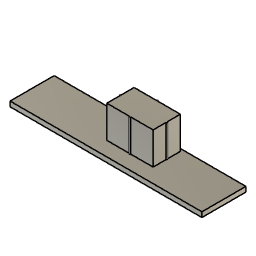
Curtains Cap (Autodesk Fusion 360 design; units mm, degrees)
Autodesk Fusion 360 part; units mm, degrees
note: some values were not read from the file. Set by a fixed rule: which sketch regions a step uses.
sketch "Sketch1" plane through (0, 0, 0) normal (0, 0, 1) x (1, 0, 0)
  line L0 (77.5, 0) -> (77.5, 17.8)
  line L1 (0, 17.8) -> (0, 0)
  line L2 (77.5, 17.8) -> (62.1, 17.8)
  line L3 (58.4, 17.8) -> (26.9, 17.8)
  line L4 (23.2, 17.8) -> (0, 17.8)
  line L5 (0, 0) -> (39.3, 0)
  line L6 (46, 0) -> (77.5, 0)
  line L7 (33.3, 5.8) -> (39.3, 5.8)
  line L8 (46, 5.8) -> (52, 5.8)
  line L9 (39.3, 0) -> (46, 0)
  line L10 (62.1, 17.8) -> (58.4, 17.8)
  line L11 (23.2, 17.8) -> (26.9, 17.8)
  arc A0 (42.95, 16.8) -> (42.35, 16.8) centre (42.65, 16.8) ccw
  line L12 (52, 16.8) -> (42.95, 16.8)
  line L13 (42.35, 16.8) -> (33.3, 16.8)
  arc A1 (33.3, 11.6) -> (33.3, 11) centre (33.3, 11.3) ccw
  line L14 (33.3, 16.8) -> (33.3, 11.6)
  line L15 (33.3, 11) -> (33.3, 5.8)
  arc A2 (42.35, 5.8) -> (42.95, 5.8) centre (42.65, 5.8) ccw
  line L16 (39.3, 5.8) -> (42.35, 5.8)
  line L17 (42.95, 5.8) -> (46, 5.8)
  arc A3 (52, 11) -> (52, 11.6) centre (52, 11.3) ccw
  line L18 (52, 5.8) -> (52, 11)
  line L19 (52, 11.6) -> (52, 16.8)
  dimension "d1" = 77.5
  dimension "d2" = 17.8
  dimension "d25" = 11
  dimension "d26" = 1
  dimension "d43" = 0.6
  dimension "d44" = 0.6
  dimension "d45" = 0.6
  dimension "d46" = 0.6
  constraint horizontal L5
  constraint vertical L0
  constraint horizontal L2
  constraint vertical L1
  constraint coincident L1.end L5.start
  constraint coincident L3.start L2
  constraint coincident L4.start L2
  constraint coincident L3.end L2
  constraint horizontal L7
  constraint vertical L18
  constraint horizontal L12
  constraint vertical L14
  constraint collinear L2 L3
  constraint collinear L3 L4
  constraint coincident L8.start L7
  constraint coincident L6.start L5
  constraint collinear L5 L6
  constraint collinear L7 L8
  constraint horizontal L11
  constraint coincident A0.end L12
  constraint collinear L12 L13
  constraint coincident A0.centre L12
  constraint coincident A1.end L14
  constraint collinear L14 L15
  constraint coincident A1.centre L14
  constraint coincident A2.end L16
  constraint collinear L16 L17
  constraint coincident A2.centre L16
  constraint coincident A3.end L18
  constraint collinear L18 L19
  constraint coincident A3.centre L18
  measures "d1" distance of L1.end L0.start
  measures "d2" distance of L1.end L1.start
  measures "d25" distance of L7 L12
  measures "d26" distance of L2 L12
  measures "d43" diameter of A2
  measures "d44" diameter of A1
  measures "d45" diameter of A3
  measures "d46" diameter of A0
extrude "Extrude1" add sketch "Sketch1" along normal blind 2
extrude "Extrude2" add sketch "Sketch1" along normal blind 15 contours L7 L8 A0 L12 L13 A1 L14 L15 A2 L16 L17 A3 L18 L19
sketch "Sketch2" plane through (0, 0, 0) normal (0, 0, 1) x (1, 0, 0)
  line L0 (33.3, 5.8) -> (39.3, 5.8)
  line L1 (46, 5.8) -> (52, 5.8)
  line L2 (48, 8) -> (37.3, 8)
  line L3 (37.3, 8) -> (37.3, 14.6)
  line L4 (37.3, 14.6) -> (48, 14.6)
  line L5 (48, 14.6) -> (48, 8)
  line L6 (48, 8) -> (37.3, 14.6) construction
  line L7 (37.3, 8) -> (48, 14.6) construction
  line L8 (39.3, 5.8) -> (42.35, 5.8)
  line L9 (52, 5.8) -> (52, 11)
  line L10 (33.3, 16.8) -> (33.3, 11.6)
  line L11 (52, 16.8) -> (42.95, 16.8)
  point P0 (42.65, 11.3)
  constraint horizontal L2
  constraint perpendicular L2 L3
  constraint parallel L2 L4
  constraint parallel L3 L5
  constraint coincident L6 P0
  constraint coincident L7 P0
